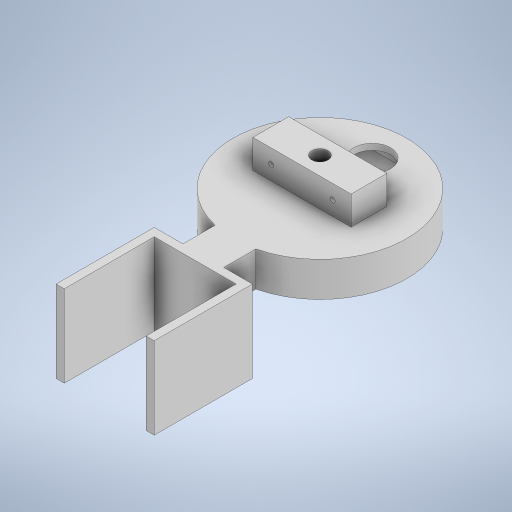
# Autodesk Inventor part: Bi_PAM_top_slot2
Saved by Autodesk Inventor 2024 (Build 280153000, 153)
## iProperties
Created: 2023-07-27
Part Number: Bi_PAM_top_slot2
Material: 일반
Document SubType Name: Modeling
Designer: jsw
Density: 1 g/cm^3
Appearance: 기본값
Author: jsw
Autodesk Inventor part; units mm, degrees
ref_plane "YZ Plane" through (0, 0, 0) normal (1, 0, 0) x (0, 1, 0)
ref_plane "XZ Plane" through (0, 0, 0) normal (0, 1, 0) x (-1, 0, 0)
ref_plane "XY Plane" through (0, 0, 0) normal (0, 0, 1) x (1, 0, 0)
sketch "스케치1" plane through (0, 0, 0) normal (0, 1, 0) x (-1, 0, 0)
  circle A0 centre (0, 0) radius 39
  circle A1 centre (0, 0) radius 42.5
  dimension "d0" = 78
  dimension "d1" = 3.5
  constraints: 2 centre point, 2 coincident
  measures "d0" diameter of A0
  measures "d1" radial gap between concentric circles of A0 A1
extrude "돌출1" add sketch "스케치1" along normal blind 7 contours A0 | A1
sketch "스케치2" plane through (0, 0, 0) normal (0, -1, 0) x (1, 0, 0)
  line L0 (15, -36.2132) -> (-15, -36.2132)
  line L1 (-15, -36.2132) -> (-36.2132, -15)
  line L2 (-36.2132, -15) -> (-36.2132, 15)
  line L3 (-36.2132, 15) -> (-15, 36.2132)
  line L4 (-15, 36.2132) -> (15, 36.2132)
  line L5 (15, 36.2132) -> (36.2132, 15)
  line L6 (36.2132, 15) -> (36.2132, -15)
  line L7 (36.2132, -15) -> (15, -36.2132)
  point P0 (0, 0)
  point P1 (0, 0)
  dimension "d5" = 30
  constraints: 16 end point, 1 coincident, 1 horizontal, 17 other
  measures "d5" distance of L5.end L6.end
extrude "돌출2" cut sketch "스케치2" against normal blind 4
fillet "모깎기1" radius 1.2 8 edges at (0, 4, 36.2132) (-25.6066, 4, 25.6066) (25.6066, 4, 25.6066) (36.2132, 4, 0) (25.6066, 4, -25.6066) (0, 4, -36.2132) (-25.6066, 4, -25.6066) (-36.2132, 4, 0)
sketch "스케치3" plane through (0, 0, 0) normal (0, -1, 0) x (1, 0, 0)
  line L0 (-15, 36.2132) -> (15, 36.2132) projected
  circle A0 centre (0, 0) radius 39.1969
  circle A1 centre (0, 0) radius 41.1969
  dimension "d9" = 2
  constraints: 2 coincident, 1 centre point, 3 other
extrude "돌출3" cut sketch "스케치3" against normal blind 4
sketch "스케치4" plane through (0, 7, 0) normal (0, 1, 0) x (1, 0, 0)
  line L0 (-24, 8.75) -> (24, 8.75)
  line L1 (24, 8.75) -> (24, -8.75)
  line L2 (24, -8.75) -> (-24, -8.75)
  line L3 (-24, -8.75) -> (-24, 8.75)
  point P0 (0, 0)
  point P1 (0, 8.75)
  point P2 (24, 0)
  dimension "d12" = 48
  dimension "d13" = 17.5
  constraints: 8 end point, 2 midpoint, 2 parallel, 1 horizontal, 1 horizontal alignment, 1 perpendicular, 1 vertical alignment
  measures "d12" distance of L0.start L0.end
  measures "d13" distance of L0.end L1.end
extrude "돌출4" add sketch "스케치4" along normal blind 14
sketch "스케치6" plane through (0, 4, 0) normal (0, -1, 0) x (1, 0, 0)
  line L0 (10, -2.75) -> (21, -2.75)
  line L1 (21, -2.75) -> (21, 2.75)
  line L2 (21, 2.75) -> (10, 2.75)
  line L3 (10, 2.75) -> (10, -2.75)
  line L4 (10, -2.75) -> (21, 2.75) construction
  line L5 (21, -2.75) -> (10, 2.75) construction
  line L6 (-10, -2.5) -> (-21, -2.5)
  line L7 (-21, -2.5) -> (-21, 2.5)
  line L8 (-21, 2.5) -> (-10, 2.5)
  line L9 (-10, 2.5) -> (-10, -2.5)
  line L10 (-10, -2.5) -> (-21, 2.5) construction
  line L11 (-21, -2.5) -> (-10, 2.5) construction
  point P0 (0, 0)
  point P1 (15.5, 0)
  point P2 (-15.5, 0)
  point P3 (-10, 0)
  dimension "d16" = 11
  dimension "d17" = 5.5
  dimension "d18" = 11
  dimension "d19" = 5
  dimension "d20" = 10
  dimension "d21" = 10
  constraints: 24 end point, 5 midpoint, 4 parallel, 2 horizontal, 2 horizontal alignment, 2 perpendicular
  measures "d16" distance of L2.end L1.end
  measures "d17" distance of L1.end L0.end
  measures "d18" distance of L7.end L8.end
  measures "d19" distance of L6.end L7.end
  measures "d20" distance from line of point (0, 0) L3
  measures "d21" distance of point (-10, 0) point (0, 0)
extrude "돌출5" cut sketch "스케치6" against normal blind 14
sketch "스케치7" plane through (0, 21, 0) normal (0, 1, 0) x (1, 0, 0)
  circle A0 centre (0, 0) radius 4
  dimension "d24" = 8
  constraints: 1 centre point, 1 coincident
  measures "d24" diameter of A0
extrude "돌출6" cut sketch "스케치7" against normal up to surface (17 mm away)
sketch "스케치8" plane through (-24, 7, 8.75) normal (0, 0, 1) x (1, 0, 0)
  circle A0 centre (9, 7) radius 1.25
  circle A1 centre (39, 7) radius 1.25
  line L0 (66.5, 0) -> (-18.5, 0) projected
  line L1 (24, 0) -> (24, 14)
  line L2 (20, 14) -> (28, 14) projected
  point P0 (24, -7)
  dimension "d27" = 2.5
  dimension "d28" = 2.5
  dimension "d30" = 15
  dimension "d31" = 15
  dimension "d32" = 7
  dimension "d33" = 7
  constraints: 2 centre point, 2 end point, 2 midpoint
  measures "d27" diameter of A0
  measures "d28" diameter of A1
  measures "d30" distance from line of L1 A1.centre
  measures "d31" distance from line of A0.centre L1
  measures "d32" distance from line of L0 A1.centre
  measures "d33" distance from line of L0 A0.centre
extrude "돌출7" cut sketch "스케치8" against normal up to surface (17.5 mm away)
sketch "스케치9" plane through (0, 7, 0) normal (0, 1, 0) x (1, 0, 0)
  line L0 (24, 8.75) -> (-24, 8.75) projected
  circle A0 centre (0, 0) radius 25.5453
  circle A1 centre (0, 25.5453) radius 9
  dimension "d36" = 18
  constraints: 2 centre point, 2 point on circle, 1 coincident, 1 vertical alignment
  measures "d36" diameter of A1
extrude "돌출8" cut sketch "스케치9" against normal up to surface (3 mm away) contours A1 A0 | A0 A1
chamfer "모따기1" distance 1 angle 45 9 edges at (15.5, 4, -2.75) (21, 4, 0) (15.5, 4, 2.75) (10, 4, 0) (-10, 4, 0) (-15.5, 4, -2.5) (-15.5, 4, 2.5) (-21, 4, 0) (-4, 4, 0)
sketch "스케치10" plane through (0, 0, 0) normal (0, -1, 0) x (1, 0, 0)
  circle A0 centre (0, 0) radius 41.1969 projected
  circle A1 centre (0, 0) radius 42.5 projected
extrude "돌출9" add sketch "스케치10" along normal blind 10
sketch "스케치11" plane through (0, 7, 0) normal (0, 1, 0) x (1, 0, 0)
  line L0 (-10, -61) -> (10, -61)
  line L1 (10, -61) -> (10, -41)
  line L2 (10, -41) -> (-10, -41)
  line L3 (-10, -41) -> (-10, -61)
  line L4 (-10, -61) -> (10, -41) construction
  line L5 (10, -61) -> (-10, -41) construction
  circle A0 centre (0, 0) radius 42.5 projected
  point P0 (0, -51)
  point P1 (10, -41.3068)
  point P2 (-10, -41.3068)
  dimension "d44" = 10
  dimension "d45" = 20
  dimension "d49" = 41
  constraints: 12 end point, 2 midpoint, 2 parallel, 1 horizontal, 1 perpendicular, 1 vertical alignment
  measures "d44" distance from line of point (0, -51) L1
  measures "d45" distance of L0.end L1.end
  measures "d49" distance from line of L2 point (0, 0)
extrude "돌출10" add sketch "스케치11" against normal up to surface (17 mm away) contours L3 A0 L1 L0
sketch "스케치12" plane through (0, 7, 0) normal (0, 1, 0) x (1, 0, 0)
  line L0 (20, -101) -> (-20, -101)
  line L1 (-20, -101) -> (-20, -61)
  line L2 (-20, -61) -> (20, -61)
  line L3 (20, -61) -> (20, -101)
  line L4 (20, -101) -> (-20, -61) construction
  line L5 (-20, -101) -> (20, -61) construction
  line L6 (24, -105) -> (-24, -105)
  line L7 (-24, -105) -> (-24, -57)
  line L8 (-24, -57) -> (24, -57)
  line L9 (24, -57) -> (24, -105)
  line L10 (24, -105) -> (-24, -57) construction
  line L11 (-24, -105) -> (24, -57) construction
  line L12 (-10, -61) -> (10, -61) projected
  line L13 (-20, -101) -> (-20, -105)
  line L14 (20, -101) -> (20, -105)
  point P0 (0, 0)
  point P1 (0, -81)
  point P2 (0, -61)
  dimension "d50" = 40
  dimension "d51" = 40
  dimension "d52" = 4
  dimension "d53" = 20
  constraints: 28 end point, 5 midpoint, 4 parallel, 4 perpendicular, 3 point on line, 2 horizontal, 1 vertical alignment
  measures "d50" distance of L1.end L2.end
  measures "d51" distance of L2.end L0.start
  measures "d52" distance between parallel lines of L2 L8
  measures "d53" distance of point (0, -61) point (0, -81)
extrude "돌출11" add sketch "스케치12" against normal blind 40 contours L3 L2 L1 L13 L6 L7 L8 L9 L14
sketch "스케치13" plane through (-24, 7, 57) normal (-1, 0, 0) x (0, 0, 1)
  point P0 (-57, -7)
